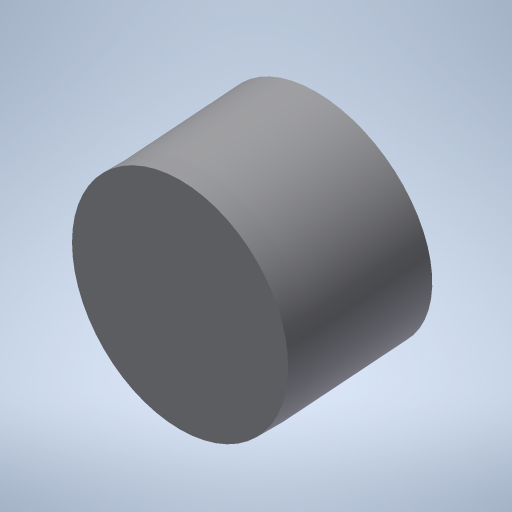
# Autodesk Inventor part: cable medio, anular
Saved by Autodesk Inventor 2023 (Build 270158000, 158)
## iProperties
Created: 2022-10-18
Part Number: cable medio, anular
Material: Generic
Document SubType Name: Modeling
Designer: Xiaba
Density: 1 g/cm^3
Appearance: Default
Author: Xiaba
Autodesk Inventor part; units mm, degrees
ref_plane "YZ Plane" through (0, 0, 0) normal (1, 0, 0) x (0, 1, 0)
ref_plane "XZ Plane" through (0, 0, 0) normal (0, 1, 0) x (-1, 0, 0)
ref_plane "XY Plane" through (0, 0, 0) normal (0, 0, 1) x (1, 0, 0)
sketch "Sketch1" plane through (0, 0, 0) normal (1, 0, 0) x (0, 1, 0)
  line L0 (0, 0) -> (0, -0.1)
  line L1 (0, -0.1) -> (0.037, -0.5986)
  dimension "d7" = 0.1
  dimension "d15" = 0.5
  constraints: 4 end point, 1 vertical
  measures "d7" distance of L0.start L0.end
  measures "d15" distance of L0.end L1.end
sketch "Sketch2" plane through (0, 0, 0) normal (0, 0, 1) x (1, 0, 0)
  circle A0 centre (0, 0) radius 0.45
  dimension "d1" = 0.9
  constraints: 1 centre point, 1 coincident
  measures "d1" diameter of A0
sweep "Sweep4" add profiles "Sketch2" path "Sketch1"
sketch "Sketch3" plane through (0, 0, 0) normal (0, 1, 0) x (-1, 0, 0)
  ellipse E0 centre (0, -0.5986) end of major axis (-0.45, -0.5986) minor radius 0.0333 projected
  line L0 (0, -0.5986) -> (2.9723, -7.0817)
  line L1 (0, -0.5986) -> (0, -5.327)
  point P0 (0, 0)
  dimension "d18" = 24.63
  dimension "d19" = 7.132
  constraints: 4 end point, 1 vertical, 1 other
  measures "d18" angle of L1 L0
  measures "d19" distance of L0.start L0.end
body "Solid4"
